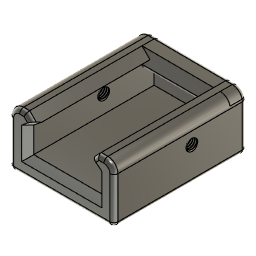
strip bumper v1 (Autodesk Fusion 360 design; units mm, degrees)
Autodesk Fusion 360 part; units mm, degrees
sketch "plate" plane through (0, 0, 0) normal (0, 0, 1) x (1, 0, 0) in component "strip clamp v18"
  line L0 (0, 0) -> (26, 0)
  line L1 (26, 0) -> (26, 4)
  line L2 (26, 4) -> (0, 4)
  line L3 (0, 4) -> (0, 0)
  line L4 (26, 0) -> (22, 0)
  line L5 (22, 0) -> (22, 10.4)
  line L6 (22, 10.4) -> (26, 10.4)
  line L7 (26, 10.4) -> (26, 0)
  line L8 (0, 0) -> (0, 10.4)
  line L9 (0, 10.4) -> (4, 10.4)
  line L10 (4, 10.4) -> (4, 0)
  line L11 (4, 0) -> (0, 0)
  line L12 (22, 10.4) -> (20, 12)
  line L13 (20, 12) -> (21.8484, 13.9014)
  line L14 (21.8484, 13.9014) -> (26, 13.9014)
  line L15 (26, 13.9014) -> (26, 10.4)
  line L16 (4, 10.4) -> (6, 12)
  line L17 (6, 12) -> (4, 14)
  line L18 (4, 14) -> (0, 14)
  line L19 (0, 14) -> (0, 10.4)
  dimension "d22" = 26
  dimension "d23" = 4
  dimension "d24" = 4
  dimension "d25" = 10.4
  dimension "d26" = 4
  dimension "d27" = 10.4
  dimension "d52" = 6
  dimension "d54" = 6
  dimension "d55" = 1.6
  dimension "d56" = 1.6
  constraint horizontal L0
  constraint vertical L1
  constraint horizontal L2
  constraint vertical L3
  constraint coincident L0.start L3.end
  constraint horizontal L4
  constraint vertical L5
  constraint horizontal L6
  constraint vertical L7
  constraint horizontal L11
  constraint vertical L8
  constraint horizontal L9
  constraint vertical L10
  constraint perpendicular L5 L14
  constraint perpendicular L10 L18
  constraint perpendicular L9 L19
  constraint perpendicular L6 L15
  measures "d22" distance of L0.start L0.end
  measures "d23" distance of L0.start L2.end
  measures "d24" distance of L0.end L4.end
  measures "d25" distance of L0.end L6.end
  measures "d26" distance of L10.end L0.start
  measures "d27" distance of L10.end L9.end
  measures "d52" distance of L16.end L19
  measures "d54" distance of L12.end L15
  measures "d55" distance of L6 L12.end
  measures "d56" distance of L9 L16.end
extrude "Extrude2" add sketch "plate" along normal blind 80 makes body 1 in component "strip clamp v18"
fillet "Fillet1" radius 2 1 edges at (0, 14, 40) on bodies 1 in component "strip clamp v18"
chamfer "Chamfer1" distance 1 distance2 2 5 edges at (5, 11.2, 80) (4, 7.2, 80) (13, 4, 80) (22, 7.2, 80) (21, 11.2, 80) measured on face at (10, 1.3333, 80) measured on face at (10, 1.3333, 80) measured on face at (10, 1.3333, 80) measured on face at (10, 1.3333, 80) measured on face at (10, 1.3333, 80) on bodies 1 in component "strip clamp v18"
move_body "Move1" bodies 1 to x (1, 0, 0) y (0, 0, 1) z (0, -1, 0) at (0, 6.5916, 6.5916) in component "strip clamp v18"
move_body "Align1" bodies 1 to x (1, 0, 0) y (0, 1, 0) z (0, 0, 1) at (0, 0, -6.5916) in component "strip clamp v18"
hole "Hole3" at (26, -53.8767, 8.4977) direction (-1, 0, 0) diameter 2.529 depth 27 tip angle 180 bodies 1 in component "strip clamp v18"
thread "Thread3" "ISO Metric profile 3.0 M3x0.5 6H" major diameter 3.086 minor diameter 2.529 pitch 0.5 angle 60 modelled right hand crest width 0.1368 on face at (24.6667, -53.7508, 9.756) crest through (25.875, -52.6122, 8.4977) on face at (2.6667, -53.8136, 9.7607) crest through (3.875, -52.6122, 8.4977) on bodies 1 in component "strip clamp v18"
fillet "Fillet3" radius 2.5 1 edges at (26, -33.4084, 13.9014) on bodies 1 in component "strip clamp v18"
delete_face "DeleteFace3" 1 faces at (0.0023, -20.0751, 12.0952) on bodies 1 in component "strip clamp v18"
fillet "Fillet4" radius 2.5 1 edges at (0, -33.4084, 14) on bodies 1 in component "strip clamp v18"
hole "Hole1" [suppressed] in component "strip clamp v18"
thread "Thread1" [suppressed] in component "strip clamp v18"
hole "Hole2" [suppressed] in component "strip clamp v18"
thread "Thread2" [suppressed] in component "strip clamp v18"
extrude "Extrude1" [suppressed] in component "strip clamp v18"
move_face "OffsetFaces1" offset -51 1 faces at (10, 6.5916, 1.3333) on bodies 1 in component "strip clamp v18"
sketch "Sketch1" plane through (0, -44.4084, 0) normal (0, 1, 0) x (-1, 0, 0)
  arc A0 (0, 11.5) -> (-2.5, 14) centre (-2.5, 11.5) ccw
  line L0 (-2.5, 14) -> (-4, 14)
  line L1 (-4, 14) -> (-6, 12)
  line L2 (-6, 12) -> (-4, 10.4)
  line L3 (-4, 10.4) -> (-4, 4)
  line L4 (-4, 4) -> (-22, 4)
  line L5 (-22, 4) -> (-22, 10.4)
  line L6 (-22, 10.4) -> (-20, 12)
  line L7 (-20, 12) -> (-21.8484, 13.9014)
  line L8 (-21.8484, 13.9014) -> (-23.5, 13.9014)
  arc A1 (-23.5, 13.9014) -> (-26, 11.4014) centre (-23.5, 11.4014) ccw
  line L9 (-26, 11.4014) -> (-26, 0)
  line L10 (-26, 0) -> (0, 0)
  line L11 (0, 0) -> (0, 11.5)
  line L12 (-21.8484, 13.9014) -> (-23.5, 13.9014)
  arc A2 (-23.5, 13.9014) -> (-25.9385, 11.9525) centre (-23.5, 11.4014) ccw
  line L13 (-26, 0) -> (0, 0)
  line L14 (-2.5, 14) -> (-2.4218, 14)
  line L15 (-2.4218, 14) -> (-4, 14)
  line L16 (-4, 14) -> (-21.8484, 13.9014)
  constraint coincident L7.end L8.start
  constraint perpendicular L9 L12
  constraint coincident A1 A2.end
  constraint tangent L12 A2
  constraint coincident L9.end L10.start
  constraint coincident L10.end L11.start
  constraint coincident A0 L0.start
  constraint tangent A0 L14
  constraint coincident L0.end L1.start
  constraint parallel L0 L15
extrude "Extrude3" add sketch "Sketch1" along normal blind 4 bodies 1 in component "strip clamp v18"
copy_body "CutPasteBodies1" bodies 1 removing the originals makes body 2
fillet "Fillet1'" radius 1 9 edges at (12.9242, -40.4084, 13.9507) (22.6742, -40.4084, 13.9014) (25.0608, -40.4084, 13.3543) (25.9846, -40.4084, 11.6787) (26, -40.4084, 5.7007) (0, -40.4084, 5.75) (0.7322, -40.4084, 13.2678) (3.25, -40.4084, 14) (13, -40.4084, 0) on bodies 2
fillet "Fillet2" radius 1 13 edges at (13, -73.4084, 0) (25.7071, -40.7013, 0.2929) (26, -57.4084, 0) (0.2929, -40.7013, 0.2929) (0, -57.4084, 0) (3.25, -73.4084, 14) (0.7322, -73.4084, 13.2678) (0, -73.4084, 5.75) (26, -73.4084, 5.7007) (25.2678, -73.4084, 13.1692) (22.6742, -73.4084, 13.9014) (4.6443, -73.4084, 13.3557) (21.2744, -73.4084, 13.3109) on bodies 2
sketch "Sketch2" plane through (0, -44.4084, 0) normal (0, -1, 0) x (1, 0, 0)
  line L0 (20, 12) -> (21.8484, 13.9014)
  line L1 (21.8484, 13.9014) -> (4, 14)
  line L2 (4, 14) -> (6, 12)
  line L3 (6, 12) -> (4, 10.4)
  line L4 (4, 10.4) -> (4, 4)
  line L5 (4, 4) -> (22, 4)
  line L6 (22, 4) -> (22, 10.4)
  line L7 (22, 10.4) -> (20, 12)
  line L8 (4, 9) -> (22, 9)
  line L9 (22, 9) -> (22, 4)
  line L10 (22, 4) -> (4, 4)
  line L11 (4, 4) -> (4, 9)
  dimension "d15" = 5
  constraint horizontal L8
  constraint vertical L9
  constraint horizontal L10
  constraint vertical L11
  constraint coincident L5.end L6.start
  measures "d15" distance of L8 L10
extrude "Extrude1'" cut sketch "Sketch2" against normal blind 3 contours L4 L5 L6 L8 L9 L10 L11 bodies 2
fillet "Fillet3'" radius 1 1 edges at (13, -44.4084, 9) on bodies 2
component "strip clamp v18" placed x (1, 0, 0) y (0, 1, 0) z (0, 0, 1) at (0, 0, 0)
